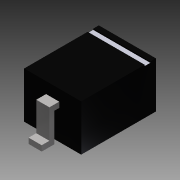
# Autodesk Inventor part: s0.57A 10V Diode
Saved by Autodesk Inventor 2015 (Build 190159000, 159)
## iProperties
Created: 2016-01-19
Part Number: s0.57A 10V Diode
Material: Generic
Document SubType Name: Modeling
Designer: Kyle
Density: 1 g/cm^3
Appearance: Default
Author: Kyle
Autodesk Inventor part; units mm, degrees
ref_plane "YZ Plane" through (0, 0, 0) normal (1, 0, 0) x (0, 1, 0)
ref_plane "XZ Plane" through (0, 0, 0) normal (0, 1, 0) x (-1, 0, 0)
ref_plane "XY Plane" through (0, 0, 0) normal (0, 0, 1) x (1, 0, 0)
sketch "Sketch1" plane through (0, 0, 0) normal (0, 0, 1) x (1, 0, 0)
  line L0 (0, 0) -> (1.3005, 0)
  line L1 (1.3005, 0) -> (1.3005, 1.049)
  line L2 (1.3005, 1.049) -> (0, 1.049)
  line L3 (0, 1.049) -> (0, 0)
  dimension "d0" = 1.049
  dimension "d1" = 1.3005
  constraints: 8 end point, 2 parallel, 1 horizontal, 1 perpendicular
  measures "d0" distance of L0.end L1.end
  measures "d1" distance of L1.end L2.end
extrude "Extrusion1" add sketch "Sketch1" along normal blind 1.7018
sketch "Sketch2" plane through (0, 0, 1.7018) normal (0, 0, 1) x (1, 0, 0)
  line L0 (0.5004, 0.795) -> (0.8001, 0.795)
  line L1 (0.8001, 0.795) -> (0.8001, 0.6706)
  line L2 (0.8001, 0.6706) -> (0.5004, 0.6706)
  line L3 (0.5004, 0.6706) -> (0.5004, 0.795)
  line L4 (0, 1.049) -> (0, 0) projected
  line L5 (1.3005, 1.049) -> (0, 1.049) projected
  dimension "d4" = 0.2997
  dimension "d5" = 0.5004
  dimension "d6" = 0.254
  dimension "d7" = 0.1245
  constraints: 8 end point, 2 parallel, 1 horizontal, 1 perpendicular
  measures "d4" distance of L0.start L0.end
  measures "d5" distance between parallel lines of L4 L3
  measures "d6" distance between parallel lines of L5 L0
  measures "d7" distance between parallel lines of L0 L2
extrude "Extrusion2" add sketch "Sketch2" against normal blind 1.8009
extrude "Extrusion3" add sketch "Sketch2" along normal blind 0.0991
sketch "Sketch3" plane through (0, 0, 1.8009) normal (0, 0, 1) x (1, 0, 0)
  line L0 (0.5004, 0.795) -> (0.8001, 0.795)
  line L1 (0.8001, 0.795) -> (0.8001, 0.6706)
  line L2 (0.8001, 0.6706) -> (0.5004, 0.6706)
  line L3 (0.5004, 0.6706) -> (0.5004, 0.795)
  point P0 (0, 0)
  constraints: 8 end point, 2 parallel, 1 horizontal, 1 perpendicular
extrude "Extrusion4" add sketch "Sketch3" along normal blind 0.1245
sketch "Sketch4" plane through (0, 0, -0.0991) normal (0, 0, -1) x (-1, 0, 0)
  line L0 (-0.8001, 0.795) -> (-0.5004, 0.795)
  line L1 (-0.5004, 0.795) -> (-0.5004, 0.6706)
  line L2 (-0.5004, 0.6706) -> (-0.8001, 0.6706)
  line L3 (-0.8001, 0.6706) -> (-0.8001, 0.795)
  point P0 (0, 0)
  constraints: 8 end point, 2 parallel, 1 horizontal, 1 perpendicular
extrude "Extrusion5" add sketch "Sketch4" along normal blind 0.1245
sketch "Sketch5" plane through (0.5004, 0.6706, 0) normal (0, -1, 0) x (1, 0, 0)
  line L0 (0.2997, 0) -> (0.2997, -0.2235) projected
  line L1 (0, -0.2235) -> (0.2997, -0.2235)
  line L2 (0.2997, -0.2235) -> (0.2997, -0.1118)
  line L3 (0.2997, -0.1118) -> (0, -0.1118)
  line L4 (0, -0.1118) -> (0, -0.2235)
  line L5 (0.2997, 1.7018) -> (0.2997, 1.9253) projected
  line L6 (0, 1.9253) -> (0.2997, 1.9253)
  line L7 (0.2997, 1.9253) -> (0.2997, 1.8136)
  line L8 (0.2997, 1.8136) -> (0, 1.8136)
  line L9 (0, 1.8136) -> (0, 1.9253)
  point P0 (-0.5004, 0)
  constraints: 16 end point, 4 parallel, 2 horizontal, 2 midpoint, 2 perpendicular
extrude "Extrusion6" add sketch "Sketch5" along normal blind 0.6604
sketch "Sketch6" plane through (0, 0, -0.2235) normal (0, 0, -1) x (-1, 0, 0)
  line L0 (-0.8001, 0.795) -> (-0.8001, 0.0102) projected
  line L1 (-0.5004, 0.0102) -> (-0.8001, 0.0102)
  line L2 (-0.8001, 0.0102) -> (-0.8001, 0.1346)
  line L3 (-0.8001, 0.1346) -> (-0.5004, 0.1346)
  line L4 (-0.5004, 0.1346) -> (-0.5004, 0.0102)
  point P0 (0, 0)
  dimension "d18" = 0.1245
  constraints: 8 end point, 2 parallel, 1 horizontal, 1 perpendicular, 1 point on line
  measures "d18" distance between parallel lines of L1 L3
extrude "Extrusion7" add sketch "Sketch6" along normal blind 0.1753
sketch "Sketch7" plane through (0, 0, 1.9253) normal (0, 0, 1) x (1, 0, 0)
  line L0 (0.8001, 0.0102) -> (0.5004, 0.0102)
  line L1 (0.5004, 0.0102) -> (0.5004, 0.1346)
  line L2 (0.5004, 0.1346) -> (0.8001, 0.1346)
  line L3 (0.8001, 0.1346) -> (0.8001, 0.0102)
  point P0 (0, 0)
  constraints: 8 end point, 2 parallel, 1 horizontal, 1 perpendicular
extrude "Extrusion8" add sketch "Sketch7" along normal blind 0.1753
sketch "Sketch8" plane through (0, 1.049, 0) normal (0, 1, 0) x (1, 0, 0)
  line L0 (0, 0) -> (0, -1.7018) projected
  line L1 (0, -0.127) -> (1.3005, -0.127)
  line L2 (1.3005, -0.127) -> (1.3005, -0.254)
  line L3 (1.3005, -0.254) -> (0, -0.254)
  line L4 (0, -0.254) -> (0, -0.127)
  line L5 (1.3005, 0) -> (0, 0) projected
  line L6 (1.3005, 0) -> (1.3005, -1.7018) projected
  dimension "d23" = 0.127
  dimension "d24" = 0.127
  dimension "d25" = 0
  constraints: 8 end point, 2 parallel, 1 horizontal, 1 perpendicular, 1 point on line
  measures "d23" distance between parallel lines of L5 L1
  measures "d24" distance between parallel lines of L1 L3
  measures "d25" distance between parallel lines of L6 L2
extrude "Extrusion9" cut sketch "Sketch8" against normal blind 0.0254 contours L1 L2 L3 L0
body "Solid1"
